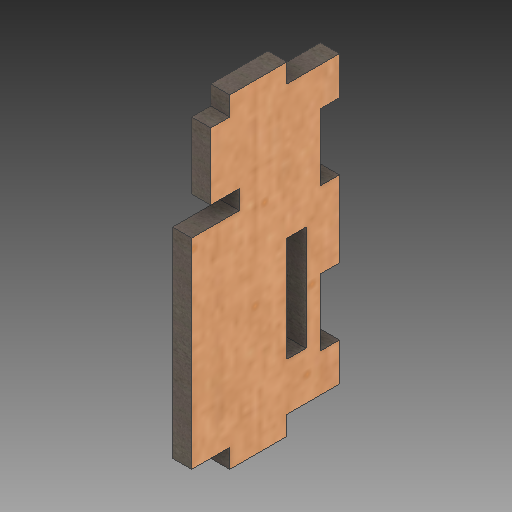
# Autodesk Inventor part: batBack
Saved by Autodesk Inventor 2019 (Build 230136000, 136)
## iProperties
Created: 2020-12-06
Part Number: batBack
Material: Дерево (береза)
Document SubType Name: Modeling
Designer: Professional
Density: 0.55 g/cm^3
Appearance: Береза — натуральный — полированный
Author: Professional
Autodesk Inventor part; units mm, degrees
ref_plane "YZ Plane" through (0, 0, 0) normal (1, 0, 0) x (0, 1, 0)
ref_plane "XZ Plane" through (0, 0, 0) normal (0, 1, 0) x (-1, 0, 0)
ref_plane "XY Plane" through (0, 0, 0) normal (0, 0, 1) x (1, 0, 0)
sketch "Эскиз2" plane through (0, 0, 0) normal (1, 0, 0) x (0, 1, 0)
  line L0 (-30, 31) -> (-30, 23)
  line L1 (-30, 23) -> (-34, 23)
  line L2 (-34, 23) -> (-34, 11)
  line L3 (-34, 11) -> (-30, 11)
  line L4 (-30, 11) -> (-30, 0)
  line L5 (-30, 0) -> (-22, 0)
  line L6 (-22, 0) -> (-22, 4)
  line L7 (-22, 4) -> (-8, 4)
  line L8 (-8, 4) -> (-8, 0)
  line L9 (-8, 0) -> (0, 0)
  line L10 (0, 0) -> (0, 31) construction
  line L11 (30, 23) -> (34, 23)
  line L12 (34, 23) -> (34, 11)
  line L13 (34, 11) -> (30, 11)
  line L14 (30, 11) -> (30, 0)
  line L15 (30, 0) -> (22, 0)
  line L16 (22, 0) -> (22, 4)
  line L17 (22, 4) -> (8, 4)
  line L18 (8, 4) -> (8, 0)
  line L19 (8, 0) -> (0, 0)
  line L20 (-20, 7) -> (2, 7)
  line L21 (2, 7) -> (2, 11)
  line L22 (2, 11) -> (-20, 11)
  line L23 (-20, 11) -> (-20, 7)
  line L24 (-30, 31) -> (12, 31)
  line L25 (12, 31) -> (12, 21)
  line L26 (12, 21) -> (16, 21)
  line L27 (16, 21) -> (16, 27)
  line L28 (16, 27) -> (30, 27)
  line L29 (30, 27) -> (30, 23)
  point P0 (0, 0)
  dimension "d0" = 4
  dimension "d1" = 12
  dimension "d2" = 8
  dimension "d4" = 11
  dimension "d5" = 60
  dimension "d6" = 14
  dimension "d7" = 16
  dimension "d8" = 10
  dimension "d9" = 22
  dimension "d10" = 7
  dimension "d13" = 42
  dimension "d15" = 10
  dimension "d16" = 4
  constraints: 60 end point, 12 perpendicular, 9 symmetric about line, 7 point on line, 3 equal length, 2 coincident, 2 horizontal, 2 parallel, 2 vertical
  measures "d0" distance of L5.end L6.end
  measures "d1" distance of L1.end L2.end
  measures "d2" distance of L0.start L0.end
  measures "d4" distance between parallel lines of L3 L5
  measures "d5" diameter of L0 L10
  measures "d6" distance between parallel lines of L8 L6
  measures "d7" diameter of L8 L10
  measures "d8" distance between parallel lines of L4 L23
  measures "d9" distance between parallel lines of L23 L21
  measures "d10" distance between parallel lines of L20 L9
  measures "d13" distance between parallel lines of L0 L25
  measures "d15" distance of L24.end L25.end
  measures "d16" distance between parallel lines of L24 L28
extrude "Выдавливание1" add sketch "Эскиз2" along normal blind 4
